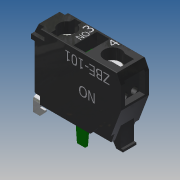
# Autodesk Inventor part: Contact NO
Saved by Autodesk Inventor 2014 (Build 180170000, 170)
## iProperties
Created: 2014-11-10
Part Number: Contact NO
Material: PPS Plastic
Document SubType Name: Modeling
Designer: David
Density: 1.637 g/cm^3
Appearance: Rubber - Black - Version 1.1
Description: CONTACT BLOCK, 1NC, 6A
Author: David
Autodesk Inventor part; units mm, degrees
ref_plane "YZ Plane" through (0, 0, 0) normal (1, 0, 0) x (0, 1, 0)
ref_plane "XZ Plane" through (0, 0, 0) normal (0, 1, 0) x (-1, 0, 0)
sketch "Sketch1" plane through (0, 0, 0) normal (0, 0, 1) x (1, 0, 0)
  line L0 (0, -3.175) -> (0, -22.0345)
  line L1 (3.175, -23.622) -> (27.2415, -23.622)
  line L2 (32.004, -10.922) -> (32.004, -3.175)
  line L3 (30.48, 0) -> (1.524, 0)
  line L4 (30.48, 0) -> (32.004, -3.175)
  line L5 (32.004, -10.922) -> (27.2415, -23.622)
  line L6 (0, -22.0345) -> (3.175, -22.0345)
  line L7 (3.175, -22.0345) -> (3.175, -23.622)
  line L8 (1.524, 0) -> (0, -3.175)
  point P0 (0, 0)
  dimension "d2" = 1.524
  dimension "d3" = 3.175
  dimension "d4" = 12.7
  dimension "d5" = 4.7625
  dimension "d6" = 32.004
  dimension "d7" = 3.175
  dimension "d8" = 1.5875
  dimension "d9" = 23.622
  constraints: 18 end point, 3 perpendicular, 2 parallel, 2 point on line, 1 equal length, 1 horizontal alignment, 1 vertical
  measures "d2" horizontal distance of L3.start L2.end
  measures "d3" vertical distance of L3.start L2.end
  measures "d4" vertical distance of L2.start L1.end
  measures "d5" horizontal distance of L2.start L1.end
  measures "d6" distance between parallel lines of L2 L0
  measures "d7" distance of L0.end L6.end
  measures "d8" distance of L1.start L6.end
  measures "d9" distance between parallel lines of L1 L3
extrude "Body" add sketch "Sketch1" along normal mid plane 9.906
sketch "Sketch2" plane through (32.004, -10.922, 4.953) normal (1, 0, 0) x (0, 0, -1)
  line L0 (1.397, 8.382) -> (8.509, 8.382)
  line L1 (8.509, 8.382) -> (8.509, 0.762)
  line L2 (8.509, 0.762) -> (1.397, 0.762)
  line L3 (1.397, 0.762) -> (1.397, 8.382)
  line L4 (4.953, -17.4244) -> (4.953, 15.6464) construction
  line L5 (0, 10.922) -> (9.906, 10.922) construction
  point P0 (4.953, 10.922)
  dimension "d12" = 2.54
  dimension "d13" = 7.62
  dimension "d14" = 7.112
  constraints: 8 end point, 2 parallel, 1 horizontal, 1 perpendicular, 1 other
  measures "d12" distance between parallel lines of L0 L5
  measures "d13" distance of L0.end L1.end
  measures "d14" distance of L0.start L0.end
extrude "Extrusion2" cut sketch "Sketch2" against normal blind 2.032
sketch "Sketch3" plane through (1.524, 0, 4.953) normal (0, 1, 0) x (1, 0, 0)
  line L0 (36.8808, 4.953) -> (-7.9248, 4.953) construction
  arc A0 (24.4451, 7.3343) -> (24.4451, 2.5718) centre (22.5425, 4.953) ccw
  line L1 (-1.524, 0) -> (-1.524, 9.906) projected
  line L2 (30.48, 8.509) -> (30.48, 9.906) projected
  line L3 (12.7635, 9.144) -> (17.2085, 9.144)
  line L4 (17.2085, 9.144) -> (17.2085, 0.762)
  line L5 (17.2085, 0.762) -> (12.7635, 0.762)
  line L6 (12.7635, 0.762) -> (12.7635, 9.144)
  line L7 (28.956, 0) -> (0, 0) projected
  line L8 (28.956, 0) -> (28.956, 9.906) projected
  line L9 (0, 9.906) -> (28.956, 9.906) projected
  line L10 (27.7654, 7.3342) -> (24.4451, 7.3343)
  line L11 (24.4451, 2.5718) -> (27.7654, 2.5718)
  line L12 (27.7654, 2.5718) -> (27.7654, 7.3342)
  line L13 (4.826, 9.144) -> (7.2072, 9.144)
  line L14 (7.2072, 0.762) -> (4.826, 0.762)
  line L15 (4.826, 0.762) -> (4.826, 2.351)
  line L16 (4.826, 7.555) -> (4.826, 9.144)
  line L17 (7.2072, 9.144) -> (7.2072, 7.8958)
  line L18 (7.2072, 2.0102) -> (7.2072, 0.762)
  arc A1 (4.826, 7.555) -> (4.826, 2.351) centre (6.4135, 4.953) ccw
  arc A2 (7.2072, 2.0102) -> (7.2072, 7.8958) centre (6.4135, 4.953) ccw
  point P0 (-1.524, 4.953)
  dimension "d17" = 6.096
  dimension "d18" = 7.9375
  dimension "d19" = 7.9375
  dimension "d20" = 8.382
  dimension "d21" = 4.445
  dimension "d22" = 14.2875
  dimension "d33" = 1.1906
  dimension "d34" = 4.7625
  dimension "d35" = 0.762
  dimension "d36" = 0.762
  dimension "d38" = 2.3813
  constraints: 26 end point, 8 parallel, 6 point on circle, 3 centre point, 3 horizontal, 3 perpendicular, 2 point on line, 2 other
  measures "d17" diameter of A0
  measures "d18" distance from line of L1 A1.centre
  measures "d19" distance from line of A0.centre L2
  measures "d20" distance of L5.end L3.start
  measures "d21" distance of L3.start L3.end
  measures "d22" distance between parallel lines of L6 L1
  measures "d33" distance between parallel lines of L12 L8
  measures "d34" distance between parallel lines of L11 L10
  measures "d35" distance between parallel lines of L13 L9
  measures "d36" distance between parallel lines of L7 L14
  measures "d38" distance of L13.start L13.end
extrude "Top" cut sketch "Sketch3" against normal blind 4.318
sketch "Sketch4" plane through (0, 0, 4.953) normal (0, 0, 1) x (1, 0, 0)
  line L0 (3.175, -23.622) -> (27.2415, -23.622) projected
  line L1 (27.2415, -23.622) -> (32.004, -10.922) projected
  line L2 (30.48, 0) -> (1.524, 0) projected
  line L3 (28.4321, -20.447) -> (23.6696, -20.447)
  line L4 (23.6696, -20.447) -> (20.8915, -23.622)
  line L5 (0, -3.175) -> (0, -22.0345) projected
  line L6 (32.004, -10.922) -> (32.004, -3.175) projected
  line L7 (0, -3.175) -> (4.7625, -3.175)
  line L8 (4.7625, -3.175) -> (4.7625, -0.762)
  line L9 (4.7625, -0.762) -> (3.556, -0.762)
  arc A0 (3.556, 0) -> (3.556, -0.762) centre (3.556, -0.381) ccw
  line L10 (1.524, 0) -> (0, -3.175) projected
  line L11 (3.556, 0) -> (1.524, 0)
  line L12 (0, -3.175) -> (1.524, 0)
  line L13 (0, -22.0345) -> (3.175, -22.0345) projected
  line L14 (3.175, -22.0345) -> (3.175, -23.622) projected
  line L15 (0, -4.7625) -> (2.3813, -4.7625)
  line L16 (2.3813, -4.7625) -> (1.5875, -12.7)
  line L17 (1.5875, -12.7) -> (3.175, -21.2408)
  line L18 (3.175, -21.2408) -> (3.175, -22.0345)
  line L19 (3.175, -22.0345) -> (0, -22.0345)
  line L20 (0, -22.0345) -> (0, -4.7625)
  point P0 (0, 0)
  dimension "d25" = 3.175
  dimension "d26" = 6.35
  dimension "d27" = 4.7625
  dimension "d42" = 0.762
  dimension "d43" = 3.175
  dimension "d44" = 4.7625
  dimension "d45" = 2.3813
  dimension "d46" = 4.7625
  dimension "d47" = 1.5875
  dimension "d48" = 12.7
  dimension "d49" = 2.3813
  constraints: 26 end point, 4 collinear, 4 perpendicular, 4 point on line, 3 tangent, 2 parallel, 2 point on circle, 1 centre point
  measures "d25" distance between parallel lines of L0 L3
  measures "d26" distance of L4.end L0.end
  measures "d27" distance of L3.start L3.end
  measures "d42" distance between parallel lines of L9 L2
  measures "d43" distance edge to line of A0 L5
  measures "d44" distance between parallel lines of L8 L5
  measures "d45" distance of L15.start L15.end
  measures "d46" distance between parallel lines of L15 L2
  measures "d47" distance from line of L5 L16.end
  measures "d48" distance from line of L2 L16.end
  measures "d49" distance from line of L17.end L0
extrude "Extrusion4" cut sketch "Sketch4" against normal blind 1.27
sketch "Sketch5" plane through (1.524, -4.318, 4.953) normal (0, 1, 0) x (1, 0, 0)
  line L0 (12.7635, 0.762) -> (12.7635, 9.144) projected
  line L1 (17.2085, 9.144) -> (17.2085, 0.762) projected
  line L2 (12.7635, 9.144) -> (17.2085, 9.144)
  line L3 (17.2085, 9.144) -> (17.2085, 7.5565)
  line L4 (17.2085, 7.5565) -> (12.7635, 7.5565)
  line L5 (12.7635, 7.5565) -> (12.7635, 9.144)
  line L6 (17.2085, 0.762) -> (12.7635, 0.762)
  line L7 (12.7635, 0.762) -> (12.7635, 2.3495)
  line L8 (12.7635, 2.3495) -> (17.2085, 2.3495)
  line L9 (17.2085, 2.3495) -> (17.2085, 0.762)
  point P0 (-1.524, 4.953)
  dimension "d30" = 1.5875
  constraints: 16 end point, 4 parallel, 2 horizontal, 2 perpendicular, 2 point on line, 1 collinear
  measures "d30" distance of L4.end L0.end
extrude "Extrusion5" cut sketch "Sketch5" against normal blind 0.762 contours L0 L8 L1 L6 | L0 L2 L1 L4
sketch "Sketch6" plane through (1.524, -4.318, 4.953) normal (0, 1, 0) x (1, 0, 0)
  arc A0 (7.2072, 2.0102) -> (7.2072, 7.8958) centre (6.4135, 4.953) ccw projected
  line L0 (24.4451, 7.3343) -> (27.7654, 7.3342) projected
  arc A1 (24.4451, 7.3343) -> (24.4451, 2.5718) centre (22.5425, 4.953) ccw projected
  line L1 (27.7654, 2.5718) -> (24.4451, 2.5718) projected
  line L2 (27.7654, 7.3342) -> (27.7654, 2.5718) projected
  circle A2 centre (6.4135, 4.953) radius 2.9618
  circle A3 centre (22.5425, 4.953) radius 2.9618
  point P0 (-1.524, 4.953)
  constraints: 2 centre point, 2 coincident, 1 equal radius
extrude "Extrusion6" add sketch "Sketch6" along normal blind 0.762 contours A2 | A3
fillet "Fillet1" radius 0.508 2 edges at (4.9757, -3.556, 0) (21.1047, -3.556, 0)
mirror "Mirror1" about plane through (0, 0, 0) normal (0, 0, 1) of "Extrusion4"
ref_plane "Work Plane1" through (16.002, -10.922, 4.953) normal (1, 0, 0) x (0, 0, -1)
mirror "Mirror2" about plane through (16.002, -10.922, 4.953) normal (1, 0, 0) of "Extrusion2"
sketch "Sketch7" plane through (0, 0, 0) normal (0, 0, 1) x (1, 0, 0)
  line L0 (0, -10.16) -> (2.032, -10.16) projected
  line L1 (0, -10.16) -> (3.175, -22.0345)
  line L2 (3.175, -22.0345) -> (0, -22.0345)
  line L3 (3.175, -21.2408) -> (3.175, -23.622) construction
  line L4 (3.175, -22.0345) -> (0, -22.0345)
  line L5 (0, -22.0345) -> (0, -10.16)
  point P0 (0, 0)
  constraints: 8 end point, 2 point on line, 1 collinear, 1 perpendicular
extrude "Extrusion7" cut sketch "Sketch7" along normal mid plane 7.112
fillet "Fillet2" radius 0.508 2 edges at (0, -22.0345, 3.6195) (0, -22.0345, -3.6195)
sketch "Sketch8" plane through (3.175, -23.622, -4.953) normal (-1, 0, 0) x (0, 0, 1)
  line L0 (9.906, 2.3813) -> (9.906, 0) projected
  line L1 (8.509, 1.5875) -> (1.397, 1.5875) projected
  line L2 (0, 0) -> (0, 2.3813) projected
  line L3 (1.27, 1.5875) -> (8.636, 1.5875)
  line L4 (9.906, 0.3175) -> (9.906, -3.302)
  line L5 (9.906, -3.302) -> (9.271, -3.302)
  line L6 (9.271, -3.302) -> (9.271, 0.3175)
  line L7 (8.636, 0.9525) -> (1.27, 0.9525)
  line L8 (0.635, 0.3175) -> (0.635, -3.302)
  line L9 (0.635, -3.302) -> (0, -3.302)
  line L10 (0, -3.302) -> (0, 0.3175)
  arc A0 (1.27, 0.9525) -> (0.635, 0.3175) centre (1.27, 0.3175) ccw
  arc A1 (9.271, 0.3175) -> (8.636, 0.9525) centre (8.636, 0.3175) ccw
  arc A2 (1.27, 1.5875) -> (0, 0.3175) centre (1.27, 0.3175) ccw
  arc A3 (9.906, 0.3175) -> (8.636, 1.5875) centre (8.636, 0.3175) ccw
  line L11 (9.906, 0) -> (0, 0) projected
  point P0 (4.953, 23.622)
  point P1 (0, 1.5875)
  point P2 (9.906, 1.5875)
  dimension "d53" = 0.635
  dimension "d54" = 0.635
  dimension "d55" = 0.635
  dimension "d56" = 1.27
  dimension "d63" = 3.302
  constraints: 16 end point, 8 point on circle, 8 tangent, 6 point on line, 4 centre point, 3 parallel, 3 perpendicular, 2 collinear, 2 equal length, 2 equal radius
  measures "d53" distance of L8.end L9.end
  measures "d54" distance between parallel lines of L7 L1
  measures "d55" radius of A0
  measures "d56" radius of A2
  measures "d63" distance between parallel lines of L5 L11
extrude "Extrusion8" add sketch "Sketch8" along normal blind 2.54 contours L0 L11 L6 A1 L7 A0 L8 L2 A2 L3 L1 A3 | L4 L5 L6 L11 | L8 L9 L10 L11
sketch "Sketch9" plane through (0, 0, 4.953) normal (0, 0, 1) x (1, 0, 0)
  line L0 (3.175, -22.0345) -> (0.635, -22.0345) projected
  line L1 (3.175, -26.924) -> (3.1496, -26.924)
  line L2 (3.1496, -26.924) -> (3.1496, -22.0345)
  line L3 (3.1496, -22.0345) -> (3.175, -22.0345)
  line L4 (3.175, -22.0345) -> (3.175, -26.924)
  point P0 (0, 0)
  dimension "d59" = 0.0254
  constraints: 8 end point, 2 parallel, 1 horizontal, 1 perpendicular, 1 point on line
  measures "d59" distance between parallel lines of L4 L2
extrude "Extrusion9" cut sketch "Sketch9" against normal through all
sketch "Sketch10" plane through (0, 0, 4.953) normal (0, 0, 1) x (1, 0, 0)
  line L0 (3.1496, -26.924) -> (3.1496, -23.3045) projected
  line L1 (0.635, -26.924) -> (0.635, -23.3045) projected
  line L2 (3.1496, -26.924) -> (0.635, -26.924) projected
  line L3 (3.1496, -26.924) -> (4.953, -25.005)
  line L4 (4.953, -25.005) -> (4.953, -24.384)
  line L5 (4.953, -24.384) -> (3.1496, -24.384)
  line L6 (3.175, -21.2408) -> (3.175, -23.622) projected
  line L7 (3.175, -23.622) -> (20.8915, -23.622) projected
  line L8 (20.8915, -23.622) -> (23.6696, -20.447) projected
  line L9 (23.6696, -20.447) -> (28.4321, -20.447) projected
  line L10 (28.4321, -20.447) -> (32.004, -10.922) projected
  line L11 (32.004, -10.922) -> (32.004, -3.175) projected
  line L12 (32.004, -3.175) -> (30.48, 0) projected
  line L13 (30.48, 0) -> (3.556, 0) projected
  arc A0 (3.556, 0) -> (3.556, -0.762) centre (3.556, -0.381) ccw projected
  line L14 (3.556, -0.762) -> (4.7625, -0.762) projected
  line L15 (4.7625, -0.762) -> (4.7625, -3.175) projected
  line L16 (4.7625, -3.175) -> (0, -3.175) projected
  line L17 (0, -3.175) -> (0, -4.7625) projected
  line L18 (0, -4.7625) -> (2.3813, -4.7625) projected
  line L19 (2.3813, -4.7625) -> (1.5875, -12.7) projected
  line L20 (1.5875, -12.7) -> (3.175, -21.2408) projected
  point P0 (0, 0)
  dimension "d62" = 4.318
  dimension "d64" = 0.762
  constraints: 6 end point, 2 perpendicular, 1 point on line
  measures "d62" distance between parallel lines of L4 L1
  measures "d64" distance between parallel lines of L5 L7
extrude "Extrusion10" add sketch "Sketch10" against normal up to surface (0.635 mm away) contours L0 L5 L4 L3
mirror "Mirror3" about plane through (0, 0, 0) normal (0, 0, 1) of "Extrusion10"
sketch "Sketch11" plane through (0, 0, 0) normal (0, 0, 1) x (1, 0, 0)
  line L0 (29.2894, 0) -> (29.2894, -4.318) construction
  line L1 (28.4321, -20.447) -> (32.004, -10.922) construction
  line L2 (29.2894, -18.161) -> (29.2894, -25.2095)
  line L3 (29.2894, -25.2095) -> (30.0831, -25.2095)
  line L4 (30.0831, -25.2095) -> (30.0831, -26.0032)
  line L5 (30.0831, -26.0032) -> (27.7019, -26.0032)
  line L6 (27.7019, -26.0032) -> (26.1144, -23.622)
  line L7 (28.4321, -20.447) -> (27.2415, -23.622) construction
  line L8 (23.6696, -20.447) -> (28.4321, -20.447) construction
  line L9 (20.8915, -23.622) -> (23.6696, -20.447) construction
  line L10 (27.2415, -23.622) -> (20.8915, -23.622) construction
  line L11 (26.1144, -23.622) -> (27.2415, -23.622)
  line L12 (27.2415, -23.622) -> (29.2894, -18.161)
  point P0 (0, 0)
  dimension "d67" = 1.5875
  dimension "d68" = 2.3813
  dimension "d69" = 0.7937
  dimension "d70" = 2.3813
  dimension "d71" = 3.175
  constraints: 14 end point, 4 collinear, 2 parallel, 2 point on line, 1 perpendicular
  measures "d67" distance between parallel lines of L3 L11
  measures "d68" distance between parallel lines of L5 L10
  measures "d69" distance of L2.end L3.end
  measures "d70" distance of L4.end L5.end
  measures "d71" distance from line of L6.end L2
extrude "Extrusion11" add sketch "Sketch11" along normal mid plane 4.699
sketch "Sketch12" plane through (3.175, -23.622, -4.953) normal (0, -1, 0) x (1, 0, 0)
  line L0 (24.0665, 8.636) -> (17.7165, 8.636) projected
  line L1 (17.7165, 1.27) -> (24.0665, 1.27) projected
  line L2 (11.4819, 8.636) -> (15.1649, 8.636)
  line L3 (15.1649, 8.636) -> (15.1649, 1.27)
  line L4 (15.1649, 1.27) -> (11.4819, 1.27)
  line L5 (11.4819, 1.27) -> (11.4819, 8.636)
  point P0 (-3.175, 4.953)
  dimension "d74" = 3.683
  constraints: 8 end point, 2 collinear, 2 parallel, 1 horizontal, 1 perpendicular
  measures "d74" distance between parallel lines of L5 L3
extrude "Extrusion12" add sketch "Sketch12" along normal blind 1.5875
sketch "Sketch13" plane through (3.175, -25.2095, -4.953) normal (0, -1, 0) x (1, 0, 0)
  line L0 (11.4819, 8.636) -> (11.4819, 1.27) projected
  line L1 (15.1649, 1.27) -> (15.1649, 8.636) projected
  line L2 (11.4819, 8.636) -> (15.1649, 8.636)
  line L3 (15.1649, 8.636) -> (15.1649, 7.62)
  line L4 (15.1649, 7.62) -> (11.4819, 7.62)
  line L5 (11.4819, 7.62) -> (11.4819, 8.636)
  line L6 (15.1649, 1.27) -> (11.4819, 1.27)
  line L7 (11.4819, 1.27) -> (11.4819, 2.286)
  line L8 (11.4819, 2.286) -> (15.1649, 2.286)
  line L9 (15.1649, 2.286) -> (15.1649, 1.27)
  point P0 (-3.175, 4.953)
  dimension "d77" = 1.016
  constraints: 16 end point, 4 parallel, 2 horizontal, 2 perpendicular, 2 point on line, 1 collinear
  measures "d77" distance of L4.end L0.start
extrude "Extrusion13" add sketch "Sketch13" along normal blind 4.7625 contours L2 L1 L4 L0 | L8 L1 L6 L0
chamfer "Chamfer1" distance 4.7625 distance2 0.3969 1 edges at (18.3399, -29.972, 3.175) measured on face at (18.3399, -24.1512, 0.889)
chamfer "Chamfer2" distance 4.7625 distance2 0.3969 1 edges at (18.3399, -29.972, -3.175) measured on face at (18.3399, -24.1512, 0.889)
chamfer "Chamfer3" distance 4.7625 distance2 0.3969 1 edges at (14.6569, -29.972, 3.175) measured on face at (14.6569, -24.1512, 0.889)
chamfer "Chamfer4" distance 4.7625 distance2 0.3969 1 edges at (14.6569, -29.972, -3.175) measured on face at (14.6569, -24.1512, -0.889)
sketch "Sketch14" plane through (30.48, 0, 4.953) normal (0, 1, 0) x (1, 0, 0)
  line L0 (-19.7612, 0.9488) -> (-19.7612, 10.0183) construction
  line L1 (-19.7612, 10.0183) -> (-15.2645, 10.0183) construction
  line L2 (-15.2645, 10.0183) -> (-15.2645, 0.9488) construction
  line L3 (-15.2645, 0.9488) -> (-19.7612, 0.9488) construction
  line L4 (-20.1291, 7.4413) -> (-20.1291, 9.7286) construction
  line L5 (-20.1291, 9.7286) -> (-17.0712, 9.7286) construction
  line L6 (-17.0712, 9.7286) -> (-17.0712, 7.4413) construction
  line L7 (-17.0712, 7.4413) -> (-20.1291, 7.4413) construction
  line L8 (-11.264, 7.4413) -> (-11.264, 9.7286) construction
  line L9 (-11.264, 9.7286) -> (-8.2061, 9.7286) construction
  line L10 (-8.2061, 9.7286) -> (-8.2061, 7.4413) construction
  line L11 (-8.2061, 7.4413) -> (-11.264, 7.4413) construction
  spline S0 degree 2 poles (-19.8351, 8.4862) (-19.8351, 8.375) (-19.7808, 8.1552) (-19.7388, 8.049) knots 0 0 0 1 2 2 2
  spline S1 degree 2 poles (-19.7388, 8.049) (-19.6968, 7.9502) (-19.6079, 7.8044) (-19.5684, 7.7476) knots 0 0 0 1 2 2 2
  line L12 (-19.5684, 7.7476) -> (-19.5684, 7.7229)
  line L13 (-19.5684, 7.7229) -> (-20.0006, 7.7229)
  spline S2 degree 2 poles (-20.0006, 7.7229) (-20.0723, 7.8563) (-20.1883, 8.3133) (-20.1883, 8.5183) knots 0 0 0 1 2 2 2
  spline S3 degree 2 poles (-20.1883, 8.5183) (-20.1883, 8.7257) (-20.1044, 9.0345) (-20.0154, 9.1605) knots 0 0 0 1 2 2 2
  spline S4 degree 2 poles (-20.0154, 9.1605) (-19.9191, 9.2939) (-19.64, 9.4322) (-19.4523, 9.4322) knots 0 0 0 1 2 2 2
  spline S5 degree 2 poles (-19.4523, 9.4322) (-19.2003, 9.4322) (-18.82, 9.1012) (-18.7706, 8.869) knots 0 0 0 1 2 2 2
  line L14 (-18.7706, 8.869) -> (-18.7409, 8.869)
  spline S6 degree 2 poles (-18.7409, 8.869) (-18.7212, 8.9653) (-18.6322, 9.1852) (-18.5433, 9.279) knots 0 0 0 1 2 2 2
  spline S7 degree 2 poles (-18.5433, 9.279) (-18.4569, 9.3729) (-18.1802, 9.4915) (-17.9802, 9.4915) knots 0 0 0 1 2 2 2
  spline S8 degree 2 poles (-17.9802, 9.4915) (-17.7751, 9.4915) (-17.4269, 9.3507) (-17.2935, 9.2222) knots 0 0 0 1 2 2 2
  spline S9 degree 2 poles (-17.2935, 9.2222) (-17.1552, 9.0888) (-17.0119, 8.7109) (-17.0119, 8.4713) knots 0 0 0 1 2 2 2
  spline S10 degree 2 poles (-17.0119, 8.4713) (-17.0119, 8.2416) (-17.1231, 7.7921) (-17.1996, 7.6389) knots 0 0 0 1 2 2 2
  line L15 (-17.1996, 7.6389) -> (-17.6319, 7.6389)
  line L16 (-17.6319, 7.6389) -> (-17.6319, 7.6686)
  spline S11 degree 2 poles (-17.6319, 7.6686) (-17.538, 7.797) (-17.3651, 8.2317) (-17.3651, 8.4466) knots 0 0 0 1 2 2 2
  spline S12 degree 2 poles (-17.3651, 8.4466) (-17.3651, 8.5726) (-17.4442, 8.8245) (-17.5356, 8.9085) knots 0 0 0 1 2 2 2
  spline S13 degree 2 poles (-17.5356, 8.9085) (-17.6269, 8.99) (-17.8443, 9.0765) (-18.0098, 9.0765) knots 0 0 0 1 2 2 2
  spline S14 degree 2 poles (-18.0098, 9.0765) (-18.1753, 9.0765) (-18.3902, 8.9802) (-18.4519, 8.8937) knots 0 0 0 1 2 2 2
  spline S15 degree 2 poles (-18.4519, 8.8937) (-18.5137, 8.8073) (-18.5606, 8.5726) (-18.5606, 8.4343) knots 0 0 0 1 2 2 2
  line L17 (-18.5606, 8.4343) -> (-18.5606, 8.2614)
  line L18 (-18.5606, 8.2614) -> (-18.899, 8.2614)
  line L19 (-18.899, 8.2614) -> (-18.899, 8.3972)
  spline S16 degree 2 poles (-18.899, 8.3972) (-18.899, 8.6714) (-19.1608, 9.0172) (-19.4103, 9.0172) knots 0 0 0 1 2 2 2
  spline S17 degree 2 poles (-19.4103, 9.0172) (-19.5264, 9.0172) (-19.6919, 8.9283) (-19.7413, 8.8567) knots 0 0 0 1 2 2 2
  spline S18 degree 2 poles (-19.7413, 8.8567) (-19.7931, 8.7801) (-19.8351, 8.5924) (-19.8351, 8.4862) knots 0 0 0 1 2 2 2
  line L20 (-16.4968, 5.2217) -> (-16.4968, 4.9187)
  line L21 (-16.4968, 4.9187) -> (-18.2489, 4.0197)
  line L22 (-18.2489, 4.0197) -> (-16.4968, 4.0197)
  line L23 (-16.4968, 4.0197) -> (-16.4968, 3.7677)
  line L24 (-16.4968, 3.7677) -> (-18.5288, 3.7677)
  line L25 (-18.5288, 3.7677) -> (-18.5288, 4.1514)
  line L26 (-18.5288, 4.1514) -> (-16.92, 4.9698)
  line L27 (-16.92, 4.9698) -> (-18.5288, 4.9698)
  line L28 (-18.5288, 4.9698) -> (-18.5288, 5.2217)
  line L29 (-18.5288, 5.2217) -> (-16.4968, 5.2217)
  spline S19 degree 2 poles (-18.2967, 7.0709) (-18.1616, 7.1862) (-17.7664, 7.3147) (-17.5128, 7.3147) knots 0 0 0 1 2 2 2
  spline S20 degree 2 poles (-17.5128, 7.3147) (-17.2658, 7.3147) (-16.8657, 7.1895) (-16.7307, 7.0709) knots 0 0 0 1 2 2 2
  spline S21 degree 2 poles (-16.7307, 7.0709) (-16.5891, 6.9458) (-16.454, 6.6148) (-16.454, 6.4156) knots 0 0 0 1 2 2 2
  spline S22 degree 2 poles (-16.454, 6.4156) (-16.454, 6.2097) (-16.594, 5.8804) (-16.7307, 5.7602) knots 0 0 0 1 2 2 2
  spline S23 degree 2 poles (-16.7307, 5.7602) (-16.8657, 5.6433) (-17.2625, 5.5181) (-17.5128, 5.5181) knots 0 0 0 1 2 2 2
  spline S24 degree 2 poles (-17.5128, 5.5181) (-17.7681, 5.5181) (-18.1567, 5.6449) (-18.2967, 5.7618) knots 0 0 0 1 2 2 2
  spline S25 degree 2 poles (-18.2967, 5.7618) (-18.4317, 5.8804) (-18.5717, 6.2114) (-18.5717, 6.4156) knots 0 0 0 1 2 2 2
  spline S26 degree 2 poles (-18.5717, 6.4156) (-18.5717, 6.623) (-18.4267, 6.9557) (-18.2967, 7.0709) knots 0 0 0 1 2 2 2
  spline S27 degree 2 poles (-17.5128, 7.0331) (-17.7137, 7.0331) (-18.025, 6.9458) (-18.127, 6.8668) knots 0 0 0 1 2 2 2
  spline S28 degree 2 poles (-18.127, 6.8668) (-18.2324, 6.7861) (-18.3378, 6.5588) (-18.3378, 6.4172) knots 0 0 0 1 2 2 2
  spline S29 degree 2 poles (-18.3378, 6.4172) (-18.3378, 6.2707) (-18.2357, 6.05) (-18.127, 5.966) knots 0 0 0 1 2 2 2
  spline S30 degree 2 poles (-18.127, 5.966) (-18.0233, 5.8853) (-17.7104, 5.7997) (-17.5128, 5.7997) knots 0 0 0 1 2 2 2
  spline S31 degree 2 poles (-17.5128, 5.7997) (-17.1127, 5.7997) (-16.6879, 6.1356) (-16.6879, 6.4172) knots 0 0 0 1 2 2 2
  spline S32 degree 2 poles (-16.6879, 6.4172) (-16.6879, 6.6988) (-17.1127, 7.0331) (-17.5128, 7.0331) knots 0 0 0 1 2 2 2
  line L30 (-9.2583, 9.6248) -> (-9.2583, 9.2617)
  line L31 (-9.2583, 9.2617) -> (-8.211, 9.2617)
  line L32 (-8.211, 9.2617) -> (-8.211, 8.869)
  line L33 (-8.211, 8.869) -> (-9.2583, 8.869)
  line L34 (-9.2583, 8.869) -> (-9.2583, 7.5229)
  line L35 (-9.2583, 7.5229) -> (-9.6881, 7.5229)
  line L36 (-9.6881, 7.5229) -> (-11.259, 8.8863)
  line L37 (-11.259, 8.8863) -> (-11.259, 9.2617)
  line L38 (-11.259, 9.2617) -> (-9.5868, 9.2617)
  line L39 (-9.5868, 9.2617) -> (-9.5868, 9.6248)
  line L40 (-9.5868, 9.6248) -> (-9.2583, 9.6248)
  line L41 (-9.5868, 8.869) -> (-10.7774, 8.869)
  line L42 (-10.7774, 8.869) -> (-9.5868, 7.844)
  line L43 (-9.5868, 7.844) -> (-9.5868, 8.869)
  point P0 (-30.48, 4.953)
  constraints: 6 other
extrude "Extrusion14" cut sketch "Sketch14" against normal blind 0.0254
sketch "Sketch15" plane through (0, 0, 4.953) normal (0, 0, 1) x (1, 0, 0)
  line L0 (32.8553, -6.0454) -> (6.9418, -6.0454) construction
  line L1 (6.9418, -6.0454) -> (6.9418, -1.1034) construction
  line L2 (6.9418, -1.1034) -> (32.8553, -1.1034) construction
  line L3 (32.8553, -1.1034) -> (32.8553, -6.0454) construction
  line L4 (32.8553, -14.3486) -> (6.9418, -14.3486) construction
  line L5 (6.9418, -14.3486) -> (6.9418, -9.4067) construction
  line L6 (6.9418, -9.4067) -> (32.8553, -9.4067) construction
  line L7 (32.8553, -9.4067) -> (32.8553, -14.3486) construction
  line L8 (25.6503, -1.9882) -> (27.8682, -1.9882)
  line L9 (27.8682, -1.9882) -> (27.8682, -2.3819)
  line L10 (27.8682, -2.3819) -> (26.1701, -4.7876)
  line L11 (26.1701, -4.7876) -> (27.791, -4.7876)
  line L12 (27.791, -4.7876) -> (27.791, -5.1632)
  line L13 (27.791, -5.1632) -> (25.6941, -5.1632)
  line L14 (25.6941, -5.1632) -> (25.6941, -4.7824)
  line L15 (25.6941, -4.7824) -> (27.4102, -2.3638)
  line L16 (27.4102, -2.3638) -> (25.6503, -2.3638)
  line L17 (25.6503, -2.3638) -> (25.6503, -1.9882)
  spline S0 degree 2 poles (23.08, -2.9633) (23.08, -2.7266) (23.2601, -2.3638) (23.4093, -2.2455) knots 0 0 0 1 2 2 2
  spline S1 degree 2 poles (23.4093, -2.2455) (23.5894, -2.1066) (23.9985, -1.9882) (24.3227, -1.9882) knots 0 0 0 1 2 2 2
  line L18 (24.3227, -1.9882) -> (25.2335, -1.9882)
  line L19 (25.2335, -1.9882) -> (25.2335, -5.1632)
  line L20 (25.2335, -5.1632) -> (24.3922, -5.1632)
  spline S2 degree 2 poles (24.3922, -5.1632) (24.0525, -5.1632) (23.7129, -5.1195) (23.5585, -5.0346) knots 0 0 0 1 2 2 2
  spline S3 degree 2 poles (23.5585, -5.0346) (23.3862, -4.9445) (23.2292, -4.6486) (23.2292, -4.4479) knots 0 0 0 1 2 2 2
  spline S4 degree 2 poles (23.2292, -4.4479) (23.2292, -4.2241) (23.4659, -3.869) (23.6743, -3.7687) knots 0 0 0 1 2 2 2
  line L21 (23.6743, -3.7687) -> (23.6743, -3.7532)
  spline S5 degree 2 poles (23.6743, -3.7532) (23.3913, -3.676) (23.08, -3.2669) (23.08, -2.9633) knots 0 0 0 1 2 2 2
  spline S6 degree 2 poles (23.5199, -2.9453) (23.5199, -3.1254) (23.6229, -3.357) (23.7772, -3.4393) knots 0 0 0 1 2 2 2
  spline S7 degree 2 poles (23.7772, -3.4393) (23.8776, -3.4908) (24.1143, -3.5217) (24.333, -3.5217) knots 0 0 0 1 2 2 2
  line L22 (24.333, -3.5217) -> (24.8116, -3.5217)
  line L23 (24.8116, -3.5217) -> (24.8116, -2.3484)
  line L24 (24.8116, -2.3484) -> (24.4694, -2.3484)
  spline S8 degree 2 poles (24.4694, -2.3484) (24.1915, -2.3484) (23.8724, -2.3999) (23.7489, -2.4822) knots 0 0 0 1 2 2 2
  spline S9 degree 2 poles (23.7489, -2.4822) (23.6306, -2.5671) (23.5199, -2.7781) (23.5199, -2.9453) knots 0 0 0 1 2 2 2
  spline S10 degree 2 poles (23.6692, -4.3887) (23.6692, -4.502) (23.7464, -4.6718) (23.8313, -4.7207) knots 0 0 0 1 2 2 2
  spline S11 degree 2 poles (23.8313, -4.7207) (23.9342, -4.7773) (24.1838, -4.803) (24.4076, -4.803) knots 0 0 0 1 2 2 2
  line L25 (24.4076, -4.803) -> (24.8116, -4.803)
  line L26 (24.8116, -4.803) -> (24.8116, -3.8742)
  line L27 (24.8116, -3.8742) -> (24.333, -3.8742)
  spline S12 degree 2 poles (24.333, -3.8742) (24.1349, -3.8742) (23.9471, -3.9153) (23.8467, -3.9797) knots 0 0 0 1 2 2 2
  spline S13 degree 2 poles (23.8467, -3.9797) (23.7489, -4.0414) (23.6692, -4.2395) (23.6692, -4.3887) knots 0 0 0 1 2 2 2
  line L28 (22.6606, -1.9882) -> (22.6606, -5.1632)
  line L29 (22.6606, -5.1632) -> (20.6743, -5.1632)
  line L30 (20.6743, -5.1632) -> (20.6743, -4.7876)
  line L31 (20.6743, -4.7876) -> (22.2386, -4.7876)
  line L32 (22.2386, -4.7876) -> (22.2386, -3.9179)
  line L33 (22.2386, -3.9179) -> (20.7798, -3.9179)
  line L34 (20.7798, -3.9179) -> (20.7798, -3.5423)
  line L35 (20.7798, -3.5423) -> (22.2386, -3.5423)
  line L36 (22.2386, -3.5423) -> (22.2386, -2.3638)
  line L37 (22.2386, -2.3638) -> (20.6743, -2.3638)
  line L38 (20.6743, -2.3638) -> (20.6743, -1.9882)
  line L39 (20.6743, -1.9882) -> (22.6606, -1.9882)
  line L40 (19.1382, -3.1846) -> (20.3398, -3.1846)
  line L41 (20.3398, -3.1846) -> (20.3398, -3.5706)
  line L42 (20.3398, -3.5706) -> (19.1382, -3.5706)
  line L43 (19.1382, -3.5706) -> (19.1382, -3.1846)
  line L44 (16.9178, -1.9882) -> (18.4667, -1.9882)
  line L45 (18.4667, -1.9882) -> (18.4667, -2.3124)
  line L46 (18.4667, -2.3124) -> (17.8904, -2.3124)
  line L47 (17.8904, -2.3124) -> (17.8904, -4.4402)
  line L48 (17.8904, -4.4402) -> (18.4667, -4.4402)
  line L49 (18.4667, -4.4402) -> (18.4667, -4.7309)
  spline S14 degree 2 poles (18.4667, -4.7309) (18.1399, -4.7309) (17.8312, -4.9162) (17.8106, -5.1735) knots 0 0 0 1 2 2 2
  line L50 (17.8106, -5.1735) -> (17.4813, -5.1735)
  line L51 (17.4813, -5.1735) -> (17.4813, -2.3124)
  line L52 (17.4813, -2.3124) -> (16.9178, -2.3124)
  line L53 (16.9178, -2.3124) -> (16.9178, -1.9882)
  spline S15 degree 2 poles (14.3577, -3.5757) (14.3577, -2.7215) (14.8543, -1.9213) (15.3715, -1.9213) knots 0 0 0 1 2 2 2
  spline S16 degree 2 poles (15.3715, -1.9213) (15.8963, -1.9213) (16.3878, -2.7369) (16.3878, -3.5731) knots 0 0 0 1 2 2 2
  spline S17 degree 2 poles (16.3878, -3.5731) (16.3878, -4.4325) (15.8912, -5.2275) (15.3715, -5.2275) knots 0 0 0 1 2 2 2
  spline S18 degree 2 poles (15.3715, -5.2275) (14.8492, -5.2275) (14.3577, -4.4042) (14.3577, -3.5757) knots 0 0 0 1 2 2 2
  spline S19 degree 2 poles (14.9032, -2.6083) (14.8414, -2.7652) (14.79, -3.2489) (14.79, -3.5757) knots 0 0 0 1 2 2 2
  spline S20 degree 2 poles (14.79, -3.5757) (14.79, -3.9025) (14.8414, -4.3836) (14.9058, -4.5457) knots 0 0 0 1 2 2 2
  spline S21 degree 2 poles (14.9058, -4.5457) (14.9701, -4.7078) (15.1939, -4.875) (15.3715, -4.875) knots 0 0 0 1 2 2 2
  spline S22 degree 2 poles (15.3715, -4.875) (15.549, -4.875) (15.778, -4.7078) (15.8449, -4.5405) knots 0 0 0 1 2 2 2
  spline S23 degree 2 poles (15.8449, -4.5405) (15.9092, -4.3785) (15.9555, -3.8845) (15.9555, -3.5731) knots 0 0 0 1 2 2 2
  spline S24 degree 2 poles (15.9555, -3.5731) (15.9555, -3.2386) (15.9144, -2.791) (15.8475, -2.616) knots 0 0 0 1 2 2 2
  spline S25 degree 2 poles (15.8475, -2.616) (15.7857, -2.4513) (15.5567, -2.2738) (15.3715, -2.2738) knots 0 0 0 1 2 2 2
  spline S26 degree 2 poles (15.3715, -2.2738) (15.1965, -2.2738) (14.9675, -2.441) (14.9032, -2.6083) knots 0 0 0 1 2 2 2
  line L54 (12.1527, -1.9882) -> (13.7016, -1.9882)
  line L55 (13.7016, -1.9882) -> (13.7016, -2.3124)
  line L56 (13.7016, -2.3124) -> (13.1253, -2.3124)
  line L57 (13.1253, -2.3124) -> (13.1253, -4.4402)
  line L58 (13.1253, -4.4402) -> (13.7016, -4.4402)
  line L59 (13.7016, -4.4402) -> (13.7016, -4.7309)
  spline S27 degree 2 poles (13.7016, -4.7309) (13.3749, -4.7309) (13.0661, -4.9162) (13.0455, -5.1735) knots 0 0 0 1 2 2 2
  line L60 (13.0455, -5.1735) -> (12.7162, -5.1735)
  line L61 (12.7162, -5.1735) -> (12.7162, -2.3124)
  line L62 (12.7162, -2.3124) -> (12.1527, -2.3124)
  line L63 (12.1527, -2.3124) -> (12.1527, -1.9882)
  line L64 (20.3076, -10.2902) -> (20.7811, -10.2902)
  line L65 (20.7811, -10.2902) -> (22.1859, -13.0278)
  line L66 (22.1859, -13.0278) -> (22.1859, -10.2902)
  line L67 (22.1859, -10.2902) -> (22.5795, -10.2902)
  line L68 (22.5795, -10.2902) -> (22.5795, -13.4652)
  line L69 (22.5795, -13.4652) -> (21.98, -13.4652)
  line L70 (21.98, -13.4652) -> (20.7013, -10.9514)
  line L71 (20.7013, -10.9514) -> (20.7013, -13.4652)
  line L72 (20.7013, -13.4652) -> (20.3076, -13.4652)
  line L73 (20.3076, -13.4652) -> (20.3076, -10.2902)
  spline S28 degree 2 poles (17.4182, -13.1024) (17.2381, -12.8914) (17.0374, -12.2739) (17.0374, -11.8777) knots 0 0 0 1 2 2 2
  spline S29 degree 2 poles (17.0374, -11.8777) (17.0374, -11.4917) (17.233, -10.8665) (17.4182, -10.6555) knots 0 0 0 1 2 2 2
  spline S30 degree 2 poles (17.4182, -10.6555) (17.6138, -10.4342) (18.1309, -10.2233) (18.4423, -10.2233) knots 0 0 0 1 2 2 2
  spline S31 degree 2 poles (18.4423, -10.2233) (18.7639, -10.2233) (19.2785, -10.442) (19.4663, -10.6555) knots 0 0 0 1 2 2 2
  spline S32 degree 2 poles (19.4663, -10.6555) (19.649, -10.8665) (19.8445, -11.4866) (19.8445, -11.8777) knots 0 0 0 1 2 2 2
  spline S33 degree 2 poles (19.8445, -11.8777) (19.8445, -12.2765) (19.6464, -12.8837) (19.4637, -13.1024) knots 0 0 0 1 2 2 2
  spline S34 degree 2 poles (19.4637, -13.1024) (19.2785, -13.3134) (18.7613, -13.5321) (18.4423, -13.5321) knots 0 0 0 1 2 2 2
  spline S35 degree 2 poles (18.4423, -13.5321) (18.1181, -13.5321) (17.5983, -13.3056) (17.4182, -13.1024) knots 0 0 0 1 2 2 2
  spline S36 degree 2 poles (17.4774, -11.8777) (17.4774, -12.1916) (17.6138, -12.6778) (17.7373, -12.8374) knots 0 0 0 1 2 2 2
  spline S37 degree 2 poles (17.7373, -12.8374) (17.8633, -13.002) (18.2184, -13.1667) (18.4397, -13.1667) knots 0 0 0 1 2 2 2
  spline S38 degree 2 poles (18.4397, -13.1667) (18.6687, -13.1667) (19.0135, -13.0072) (19.1447, -12.8374) knots 0 0 0 1 2 2 2
  spline S39 degree 2 poles (19.1447, -12.8374) (19.2707, -12.6753) (19.4045, -12.1864) (19.4045, -11.8777) knots 0 0 0 1 2 2 2
  spline S40 degree 2 poles (19.4045, -11.8777) (19.4045, -11.2524) (18.8797, -10.5886) (18.4397, -10.5886) knots 0 0 0 1 2 2 2
  spline S41 degree 2 poles (18.4397, -10.5886) (17.9997, -10.5886) (17.4774, -11.2524) (17.4774, -11.8777) knots 0 0 0 1 2 2 2
  point P0 (0, 0)
  constraints: 4 other
extrude "Extrusion15" cut sketch "Sketch15" against normal blind 0.0254
sketch "Sketch16" plane through (29.972, -10.922, 4.953) normal (1, 0, 0) x (0, 0, -1)
  line L0 (8.509, 0.762) -> (1.397, 0.762) projected
  circle A0 centre (3.175, 1.9526) radius 1.1906
  circle A1 centre (6.731, 1.9526) radius 1.1906
  line L1 (4.953, -25.0444) -> (4.953, 16.9164) construction
  point P0 (4.953, 10.922)
  dimension "d96" = 2.3813
  dimension "d99" = 3.556
  constraints: 2 centre point, 2 tangent, 1 equal radius, 1 symmetric about line
  measures "d96" diameter of A1
  measures "d99" distance of A1.centre A0.centre
extrude "Extrusion16" cut sketch "Sketch16" against normal blind 3.175
mirror "Mirror4" about plane through (16.002, -10.922, 4.953) normal (1, 0, 0) of "Extrusion16"
fillet "Fillet3" radius 0.254 8 edges at (3.175, -0.381, 4.953) (4.1593, -0.762, 4.953) (17.018, 0, 4.953) (3.175, -0.381, -4.953) (4.1593, -0.762, -4.953) (17.018, 0, -4.953) (12.0333, -23.622, 4.953) (12.0333, -23.622, -4.953)
body "Solid1"
